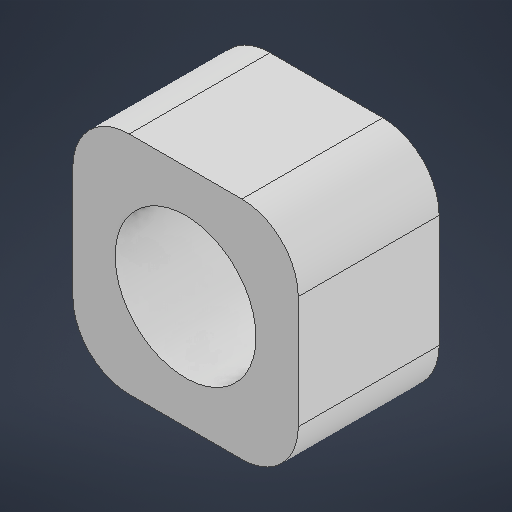
# Autodesk Inventor part: RetenedorEjeGarraVerticalSuperior
Saved by Autodesk Inventor 2026.2 (Build 302298010, 298A)
## iProperties
Created: 2026-04-22
Part Number: RetenedorEjeGarraVerticalSuperior
Material: Genérico
Document SubType Name: Modeling
Designer: Jose Carlos
Density: 1 g/cm^3
Appearance: Valor por defecto
Author: Jose Carlos
Autodesk Inventor part; units mm, degrees
ref_plane "YZ Plane" through (0, 0, 0) normal (1, 0, 0) x (0, 1, 0)
ref_plane "XZ Plane" through (0, 0, 0) normal (0, 1, 0) x (-1, 0, 0)
ref_plane "Plano de trabajo1" through (0, 0, 0) normal (0, 0, 1) x (1, 0, 0)
sketch "Boceto1" plane through (0, 0, 0) normal (0, 0, 1) x (1, 0, 0)
  arc A0 (-2.4, -0.7) -> (-0.7, -2.4) centre (0, 0) ccw construction
  circle A1 centre (0, 0) radius 2.5
  line L0 (2, 4) -> (-2, 4)
  line L1 (-4, 2) -> (-4, -2)
  line L2 (-2, -4) -> (2, -4)
  line L3 (4, -2) -> (4, 2)
  line L4 (4, 4) -> (-4, -4) construction
  line L5 (-4, 4) -> (4, -4) construction
  arc A2 (-2, 4) -> (-4, 2) centre (-2, 2) ccw
  arc A3 (4, 2) -> (2, 4) centre (2, 2) ccw
  arc A4 (-4, -2) -> (-2, -4) centre (-2, -2) ccw
  arc A5 (2, -4) -> (4, -2) centre (2, -2) ccw
  point P0 (0, 0)
  dimension "d0" = 8
  dimension "d1" = 8
  dimension "d2" = 2
  constraints: 12 end point, 8 point on circle, 8 point on line, 8 tangent, 5 centre point, 4 equal radius, 2 midpoint, 2 parallel, 1 coincident, 1 horizontal, 1 perpendicular
  measures "d0" distance of L5.start L4.end
  measures "d1" distance of L4.end L5.end
  measures "d2" radius of A2
extrude "Extrusión1" add sketch "Boceto1" along normal blind 5
